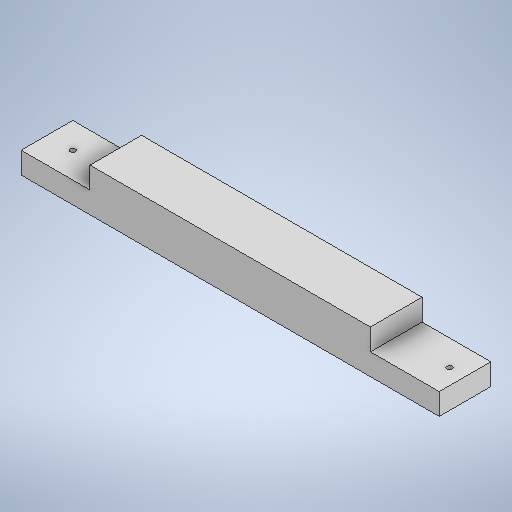
# Autodesk Inventor part: Bras_avant
Saved by Autodesk Inventor 2025.2 (Build 292293000, 293)
## iProperties
Created: 2025-03-03
Part Number: Bras_avant
Material: Générique
Document SubType Name: Modeling
Designer: Elisabete
Density: 1 g/cm^3
Appearance: Par défaut
Author: Elisabete
Autodesk Inventor part; units mm, degrees
ref_plane "YZ Plane" through (0, 0, 0) normal (1, 0, 0) x (0, 1, 0)
ref_plane "XZ Plane" through (0, 0, 0) normal (0, 1, 0) x (-1, 0, 0)
ref_plane "XY Plane" through (0, 0, 0) normal (0, 0, 1) x (1, 0, 0)
sketch "Esquisse1" plane through (0, 0, 0) normal (1, 0, 0) x (0, 1, 0)
  line L0 (0, 0) -> (25, 0)
  line L1 (25, 0) -> (25, -30)
  line L2 (25, -30) -> (0, -30)
  line L3 (0, -30) -> (0, 0)
  dimension "d0" = 25
  dimension "d1" = 30
  constraints: 8 end point, 2 parallel, 1 horizontal, 1 perpendicular
  measures "d0" distance of L1.end L2.end
  measures "d1" distance of L0.end L1.end
extrude "Extrusion1" add sketch "Esquisse1" along normal blind 243
sketch "Esquisse2" plane through (0, 25, 0) normal (0, 1, 0) x (1, 0, 0)
  circle A0 centre (15, 15) radius 1.5
  line L0 (0, 30) -> (0, 0) projected
  circle A1 centre (234, 15) radius 1.5
  dimension "d4" = 3
  dimension "d5" = 15
  dimension "d6" = 3
  dimension "d7" = 219
  constraints: 2 centre point
  measures "d4" diameter of A0
  measures "d5" distance from line of L0 A0.centre
  measures "d6" diameter of A1
  measures "d7" distance of A1.centre A0.centre
extrude "Extrusion2" cut sketch "Esquisse2" against normal blind 25 from surface at 0
sketch "Esquisse3" plane through (0, 0, 0) normal (0, 0, 1) x (1, 0, 0)
  line L0 (0, 25) -> (243, 25) projected
  line L1 (0, 25) -> (40, 25)
  line L2 (40, 25) -> (40, 12.5)
  line L3 (40, 12.5) -> (0, 12.5)
  line L4 (0, 12.5) -> (0, 25)
  line L5 (243, 25) -> (203, 25)
  line L6 (203, 25) -> (203, 12.5)
  line L7 (203, 12.5) -> (243, 12.5)
  line L8 (243, 12.5) -> (243, 25)
  point P0 (0, 0)
  dimension "d10" = 12.5
  dimension "d11" = 40
  dimension "d12" = 40
  constraints: 16 end point, 4 parallel, 2 horizontal, 2 perpendicular
  measures "d10" distance of L1.end L2.end
  measures "d11" distance of L2.end L3.end
  measures "d12" distance of L6.end L7.end
extrude "Extrusion3" cut sketch "Esquisse3" against normal through all
